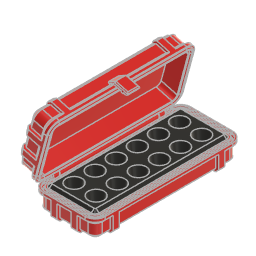
ER16 Collet Rugged Case (Autodesk Fusion 360 design; units mm, degrees)
Autodesk Fusion 360 part; units mm, degrees
note: some values were not read from the file. Chosen so that the rebuilt part matches the saved one: which face or edge a step refers to; where a step starts. Set by a fixed rule: which sketch regions a step uses.
sketch "Base Sketch" plane through (0, 0, 0) normal (0, 0, 1) x (1, 0, 0)
  line L0 (4, 0) -> (46, 0)
  line L1 (50, 4) -> (50, 131)
  line L2 (46, 135) -> (4, 135)
  line L3 (0, 131) -> (0, 4)
  arc A0 (46, 0) -> (50, 4) centre (46, 4) ccw
  arc A1 (50, 131) -> (46, 135) centre (46, 131) ccw
  arc A2 (4, 135) -> (0, 131) centre (4, 131) ccw
  arc A3 (0, 4) -> (4, 0) centre (4, 4) ccw
  point P0 (50, 0)
  point P1 (0, 135)
  dimension "d6" = 50
  dimension "d7" = 135
  dimension "d8" = 4
  constraint horizontal L0
  constraint vertical L1
  constraint horizontal L2
  constraint vertical L3
  constraint coincident P0 L0
  constraint coincident P0 L1
  constraint tangent L0 A0
  constraint tangent L1 A0
  constraint tangent L1 A1
  constraint tangent L2 A1
  constraint equal A0 A1
  constraint coincident P1 L2
  constraint coincident P1 L3
  constraint tangent L2 A2
  constraint tangent L3 A2
  constraint equal A0 A2
  constraint coincident origin L0
  constraint coincident origin L3
  constraint tangent L0 A3
  constraint tangent L3 A3
  constraint equal A0 A3
  measures "d6" distance of origin P0
  measures "d7" distance of origin P1
  measures "d8" radius of A0
ref_plane "WorkPlane1" through (0, 67.5, 0) normal (0, 1, 0) x (0, 0, 1)
sketch "Top Sketch" plane through (0, 67.5, 0) normal (0, 1, 0) x (1, 0, 0)
  line L0 (0, 0) -> (-3, 0)
  line L1 (-3, 0) -> (-3, -16.5)
  line L2 (-3, -16.5) -> (0, -16.5)
  line L3 (0, -16.5) -> (0, 0)
  line L4 (-3, -16.5) -> (-6, -16.5)
  line L5 (-6, -16.5) -> (-6, -13.5)
  line L6 (-6, -13.5) -> (-3, -13.5)
  line L7 (-3, -13.5) -> (-3, -16.5)
  line L8 (0, 0) -> (25, 0)
  line L9 (25, 0) -> (25, 3)
  line L10 (25, 3) -> (0, 3)
  line L11 (0, 3) -> (0, 0)
  line L12 (0, 3) -> (-3, 0)
  line L13 (-6, -13.5) -> (-3, -10.5)
  line L14 (-4.5, -16.5) -> (-3.3536, -17.6464)
  line L15 (-4.5, -16.5) -> (-2.3787, -16.5) construction
  line L16 (-2.6464, -17.6464) -> (-1.5, -16.5)
  arc A0 (-3.3536, -17.6464) -> (-2.6464, -17.6464) centre (-3, -17.2929) ccw
  dimension "d12" = 3
  dimension "d13" = 16.5
  dimension "d14" = 3
  dimension "d15" = 3
  dimension "d16" = 25
  dimension "d17" = 3
  dimension "d97" = 45
  dimension "d146" = 0.5
  dimension "d284" = 45
  constraint horizontal L0
  constraint vertical L1
  constraint horizontal L2
  constraint vertical L3
  constraint coincident L0.start L3.end
  constraint horizontal L4
  constraint vertical L5
  constraint horizontal L6
  constraint vertical L7
  constraint horizontal L8
  constraint vertical L9
  constraint horizontal L10
  constraint vertical L11
  constraint coincident L1 L13.end
  constraint parallel L12 L13
  constraint horizontal L15
  constraint midpoint L4 L14.start
  constraint midpoint L2 L16.end
  constraint tangent L14 A0
  constraint tangent L16 A0
  measures "d12" distance of L0.start L0.end
  measures "d13" distance of L0.start L2.end
  measures "d14" distance of L1.end L4.end
  measures "d15" distance of L1.end L6.end
  measures "d16" distance of L0.start L8.end
  measures "d17" distance of L0.start L10.end
  measures "d97" angle of L14 L15
  measures "d146" radius of A0
  measures "d284" angle of L2 L16
sweep "Sweep1" add profiles "Top Sketch" path "Base Sketch" along L0 A0 L1 A1 L2 A2 L3 A3 section 1 contours L0 L1 L2 L3 L7 | L8 L9 L10 L11 | L0 L11 L12 | L1 L6 L13 | L1 L4 L5 L6 L7 makes body 1
sketch "Bottom Sketch" plane through (0, 67.5, 0) normal (0, 1, 0) x (1, 0, 0)
  line L0 (0, 0) -> (-3, 0)
  line L1 (-3, 0) -> (-3, -16.5)
  line L2 (-3, -16.5) -> (0, -16.5)
  line L3 (0, -16.5) -> (0, 0)
  line L4 (0, 0) -> (25, 0)
  line L5 (25, 0) -> (25, 3)
  line L6 (25, 3) -> (0, 3)
  line L7 (0, 3) -> (0, 0)
  line L8 (-3, -16.5) -> (-6, -16.5)
  line L9 (-6, -16.5) -> (-6, -13.5)
  line L10 (-6, -13.5) -> (-3, -13.5)
  line L11 (-3, -13.5) -> (-3, -16.5)
  line L12 (0, 3) -> (-3, 0)
  line L13 (-6, -13.5) -> (-3, -10.5)
  line L14 (-4.5, -16.5) -> (-1.5, -16.5)
  line L15 (-1.5, -16.5) -> (-1.5, -13.5)
  line L16 (-1.5, -13.5) -> (-4.5, -13.5)
  line L17 (-4.5, -13.5) -> (-4.5, -16.5)
  line L18 (-3.3536, -13.8536) -> (-4.5, -15)
  line L19 (-2.6464, -13.8536) -> (-1.5, -15)
  arc A0 (-2.6464, -13.8536) -> (-3.3536, -13.8536) centre (-3, -14.2071) ccw
  dimension "d24" = 3
  dimension "d25" = 16.5
  dimension "d26" = 25
  dimension "d27" = 3
  dimension "d28" = 3
  dimension "d29" = 3
  dimension "d90" = 3
  dimension "d145" = 0.5
  constraint horizontal L0
  constraint vertical L1
  constraint horizontal L2
  constraint vertical L3
  constraint coincident L0.start L3.end
  constraint horizontal L4
  constraint vertical L5
  constraint horizontal L6
  constraint vertical L7
  constraint horizontal L8
  constraint vertical L9
  constraint horizontal L10
  constraint vertical L11
  constraint coincident L1 L13.end
  constraint parallel L12 L13
  constraint horizontal L14
  constraint vertical L15
  constraint horizontal L16
  constraint vertical L17
  constraint midpoint L8 L14.start
  constraint midpoint L17 L18.end
  constraint midpoint L15 L19.end
  constraint perpendicular L18 L19
  constraint coincident L10.end L18
  constraint coincident L10.end L19
  constraint tangent L18 A0
  constraint tangent L19 A0
  measures "d24" distance of L0.start L0.end
  measures "d25" distance of L0.start L2.end
  measures "d26" distance of L0.start L4.end
  measures "d27" distance of L0.start L6.end
  measures "d28" distance of L1.end L8.end
  measures "d29" distance of L1.end L10.end
  measures "d90" distance of L14.start L16.end
  measures "d145" radius of A0
sweep "Sweep2" add profiles "Bottom Sketch" path "Base Sketch" along L0 A0 L1 A1 L2 A2 L3 A3 section 1 separate body makes body 2
ref_plane "WorkPlane2" through (0, 18, 0) normal (0, 1, 0) x (0, 0, 1)
sketch "Rib Bottom" plane through (0, 18, 0) normal (0, 1, 0) x (1, 0, 0)
  line L0 (0, 0) -> (-6, 0)
  line L1 (-6, 0) -> (-6, -16.5)
  line L2 (-6, -16.5) -> (0, -16.5)
  line L3 (0, -16.5) -> (0, 0)
  line L4 (0, 0) -> (25, 0)
  line L5 (25, 0) -> (25, 3)
  line L6 (25, 3) -> (0, 3)
  line L7 (0, 3) -> (0, 0)
  line L8 (0, 0) -> (-3, 0)
  line L9 (-3, 0) -> (-3, 3)
  line L10 (-3, 3) -> (0, 3)
  line L11 (0, 3) -> (0, 0)
  line L12 (-3, 3) -> (-6, 0)
  dimension "d37" = 6
  dimension "d38" = 16.5
  dimension "d39" = 25
  dimension "d40" = 3
  dimension "d41" = 3
  dimension "d42" = 3
  constraint horizontal L0
  constraint vertical L1
  constraint horizontal L2
  constraint vertical L3
  constraint coincident L0.start L3.end
  constraint horizontal L4
  constraint vertical L5
  constraint horizontal L6
  constraint vertical L7
  constraint horizontal L8
  constraint vertical L9
  constraint horizontal L10
  constraint vertical L11
  measures "d37" distance of L0.start L0.end
  measures "d38" distance of L0.start L2.end
  measures "d39" distance of L0.start L4.end
  measures "d40" distance of L0.start L6.end
  measures "d41" distance of L0.start L8.end
  measures "d42" distance of L0.start L6.end
extrude "Extrude1" add sketch "Rib Bottom" against normal blind 6 bodies 2
ref_plane "WorkPlane3" through (0, 117, 0) normal (0, 1, 0) x (0, 0, 1)
extrude "Extrude2" add sketch "Rib Bottom" along normal blind 6 from surface at 99 bodies 2
ref_plane "WorkPlane4" through (25, 0, 0) normal (1, 0, 0) x (0, 1, 0)
mirror "Mirror1" about plane through (25, 0, 0) normal (1, 0, 0) of "Extrude1", "Extrude2"
sketch "Rib Top" plane through (0, 67.5, 0) normal (0, 1, 0) x (1, 0, 0)
  line L0 (0, 0) -> (-6, 0)
  line L1 (-6, 0) -> (-6, -16.5)
  line L2 (-6, -16.5) -> (0, -16.5)
  line L3 (0, -16.5) -> (0, 0)
  line L4 (0, 0) -> (25, 0)
  line L5 (25, 0) -> (25, 3)
  line L6 (25, 3) -> (0, 3)
  line L7 (0, 3) -> (0, 0)
  line L8 (0, 0) -> (-3, 0)
  line L9 (-3, 0) -> (-3, 3)
  line L10 (-3, 3) -> (0, 3)
  line L11 (0, 3) -> (0, 0)
  line L12 (-3, 3) -> (-6, 0)
  dimension "d52" = 6
  dimension "d53" = 16.5
  dimension "d54" = 25
  dimension "d55" = 3
  dimension "d56" = 3
  dimension "d57" = 3
  constraint horizontal L0
  constraint vertical L1
  constraint horizontal L2
  constraint vertical L3
  constraint coincident L0.start L3.end
  constraint horizontal L4
  constraint vertical L5
  constraint horizontal L6
  constraint vertical L7
  constraint horizontal L8
  constraint vertical L9
  constraint horizontal L10
  constraint vertical L11
  measures "d52" distance of L0.start L0.end
  measures "d53" distance of L0.start L2.end
  measures "d54" distance of L0.start L4.end
  measures "d55" distance of L0.start L6.end
  measures "d56" distance of L0.start L8.end
  measures "d57" distance of L0.start L6.end
extrude "Extrude3" add sketch "Rib Top" against normal blind 6 from surface at -49.5 bodies 1
extrude "Extrude4" add sketch "Rib Top" along normal blind 6 from surface at 49.5 bodies 1
mirror "Mirror2" about plane through (25, 0, 0) normal (1, 0, 0) of "Extrude3", "Extrude4"
ref_plane "WorkPlane5" through (18, 0, 0) normal (1, 0, 0) x (0, 1, 0)
ref_plane "WorkPlane6" through (32, 0, 0) normal (1, 0, 0) x (0, 1, 0)
sketch "Rib Wid" plane through (18, 0, 0) normal (1, 0, 0) x (0, 1, 0)
  line L0 (0, 0) -> (-6, 0)
  line L1 (-6, 0) -> (-6, 16.5)
  line L2 (-6, 16.5) -> (0, 16.5)
  line L3 (0, 16.5) -> (0, 0)
  line L4 (0, 0) -> (67.5, 0)
  line L5 (67.5, 0) -> (67.5, -3)
  line L6 (67.5, -3) -> (0, -3)
  line L7 (0, -3) -> (0, 0)
  line L8 (0, 0) -> (-3, 0)
  line L9 (-3, 0) -> (-3, -3)
  line L10 (-3, -3) -> (0, -3)
  line L11 (0, -3) -> (0, 0)
  line L12 (-3, -3) -> (-6, 0)
  line L13 (0, -3) -> (-6, -3)
  line L14 (-6, -3) -> (-6, 13.5)
  line L15 (-6, 13.5) -> (0, 13.5)
  line L16 (0, 13.5) -> (0, -3)
  dimension "d68" = 6
  dimension "d69" = 16.5
  dimension "d70" = 67.5
  dimension "d71" = 3
  dimension "d72" = 3
  dimension "d73" = 3
  dimension "d74" = 6
  dimension "d75" = 16.5
  constraint horizontal L0
  constraint vertical L1
  constraint horizontal L2
  constraint vertical L3
  constraint coincident L0.start L3.end
  constraint horizontal L4
  constraint vertical L5
  constraint horizontal L6
  constraint vertical L7
  constraint horizontal L8
  constraint vertical L9
  constraint horizontal L10
  constraint vertical L11
  constraint horizontal L13
  constraint vertical L14
  constraint horizontal L15
  constraint vertical L16
  measures "d68" distance of L0.start L0.end
  measures "d69" distance of L0.start L2.end
  measures "d70" distance of L0.start L4.end
  measures "d71" distance of L0.start L6.end
  measures "d72" distance of L0.start L8.end
  measures "d73" distance of L0.start L6.end
  measures "d74" distance of L6.end L13.end
  measures "d75" distance of L6.end L15.end
extrude "Extrude5" add sketch "Rib Wid" against normal blind 6 contours L0 L7 L8 L9 L10 L11 L13 L16 | L0 L1 L3 L8 L14 L15 L16 | L4 L5 L6 L7 L11 L16 | L0 L9 L12 | L1 L2 L3 L15 bodies 2
extrude "Extrude6" add sketch "Rib Wid" along normal blind 6 from surface at 14 contours L0 L7 L8 L9 L10 L11 L13 L16 | L0 L1 L3 L8 L14 L15 L16 | L4 L5 L6 L7 L11 L16 | L0 L9 L12 | L1 L2 L3 L15 bodies 2
ref_plane "WorkPlane7" through (25, 67.5, 5.25) normal (0, -1, 0) x (0, 0, -1)
mirror "Mirror3" about plane through (25, 67.5, 5.25) normal (0, -1, 0) of "Extrude5", "Extrude6"
extrude "Extrude7" add sketch "Rib Wid" against normal blind 6 contours L0 L7 L8 L9 L10 L11 L13 L16 | L0 L1 L3 L8 L14 L15 L16 | L4 L5 L6 L7 L11 L16 | L0 L9 L12 bodies 1
extrude "Extrude8" add sketch "Rib Wid" along normal blind 6 from surface at 14 contours L0 L7 L8 L9 L10 L11 L13 L16 | L0 L1 L3 L8 L14 L15 L16 | L4 L5 L6 L7 L11 L16 | L0 L9 L12 bodies 1
mirror "Mirror4" about plane through (25, 67.5, 5.25) normal (0, -1, 0) of "Extrude7", "Extrude8"
sweep "Sweep3" cut profiles "Bottom Sketch" path "Base Sketch" along L0 A0 L1 A1 L2 A2 L3 A3 section 1 contours L1 L2 L11 L14 L15 L19 A0 | L1 L8 L11 L14 L17 L18 A0 bodies 2
sweep "Sweep4" add profiles "Top Sketch" path "Base Sketch" along L0 A0 L1 A1 L2 A2 L3 A3 section 1 contours L2 L4 L14 L16 A0 bodies 1
sketch "Hinge" plane through (0, 0, 0) normal (0, 1, 0) x (1, 0, 0)
  line L0 (0, 0) -> (-6, 0) construction
  line L1 (-6, 0) -> (-6, -16.5) construction
  line L2 (-6, -16.5) -> (0, -16.5) construction
  line L3 (0, -16.5) -> (0, 0) construction
  circle A0 centre (-6, -16.5) radius 3
  circle A1 centre (-6, -16.5) radius 1.5
  circle A2 centre (-6, -16.5) radius 3.1
  line L4 (-6, -16.5) -> (-4.5, -16.5)
  line L5 (-4.5, -16.5) -> (-4.5, -19.5)
  line L6 (-4.5, -19.5) -> (-6, -19.5)
  line L7 (-6, -19.5) -> (-6, -16.5)
  line L8 (-6, -16.5) -> (-7.5, -16.5)
  line L9 (-7.5, -16.5) -> (-7.5, -19.5)
  line L10 (-7.5, -19.5) -> (-6, -19.5)
  line L11 (-6, -19.5) -> (-6, -16.5)
  line L12 (0, 0) -> (-6, 0) construction
  line L13 (-6, 0) -> (-6, -16.5) construction
  line L14 (-6, -16.5) -> (0, -16.5) construction
  line L15 (0, -16.5) -> (0, 0) construction
  circle A3 centre (-6, -16.5) radius 3
  circle A4 centre (-6, -16.5) radius 3.2
  dimension "d329" = 6
  dimension "d330" = 16.5
  dimension "d331" = 6
  dimension "d332" = 3
  dimension "d339" = 6.2
  dimension "d345" = 1.5
  dimension "d346" = 3
  dimension "d347" = 1.5
  dimension "d348" = 3
  dimension "d355" = 6
  dimension "d356" = 16.5
  dimension "d357" = 6
  dimension "d358" = 0.2
  constraint horizontal L0
  constraint vertical L1
  constraint horizontal L2
  constraint vertical L3
  constraint coincident L0.start L3.end
  constraint coincident L1.end L2.start
  constraint concentric A0 A1
  constraint concentric A0 A2
  constraint horizontal L4
  constraint vertical L5
  constraint horizontal L6
  constraint vertical L7
  constraint horizontal L8
  constraint vertical L9
  constraint horizontal L10
  constraint vertical L11
  constraint horizontal L12
  constraint vertical L13
  constraint horizontal L14
  constraint vertical L15
  measures "d329" distance of L0.start L0.end
  measures "d330" distance of L0.start L2.end
  measures "d331" diameter of A0
  measures "d332" diameter of A1
  measures "d339" diameter of A2
  measures "d345" distance of L1.end L4.end
  measures "d346" distance of L1.end L6.end
  measures "d347" distance of L1.end L8.end
  measures "d348" distance of L1.end L6.end
  measures "d355" distance of L0.start L0.end
  measures "d356" distance of L0.start L2.end
  measures "d357" diameter of A3
extrude "Extrude58" add sketch "Hinge" along normal up to surface (6 mm away) from surface at 12 contours A0 A1 L5 L9 A3 | A0 A1 L7 L9 L11 A3 | A0 A1 L5 L7 L11 A3 | A1 L7 L8 L11 | A1 L4 L8 | A1 L4 L7 L11 bodies 1
extrude "Extrude59" add sketch "Hinge" along normal up to surface (6 mm away) from surface at 117 contours A0 A1 L5 L9 A3 | A0 A1 L7 L9 L11 A3 | A0 A1 L5 L7 L11 A3 | A1 L7 L8 L11 | A1 L4 L8 | A1 L4 L7 L11 bodies 1
extrude "Extrude60" cut sketch "Hinge" along normal up to surface (99 mm away) from surface at 18 contours A0 A1 L5 L9 A3 | A0 A2 L5 L9 A3 | A0 A1 L7 L9 L11 A3 | A0 A2 L9 L10 A3 | A0 A2 L5 L6 A3 | A0 A1 L5 L7 L11 A3 | A2 L6 L10 | A1 L7 L8 L11 | A1 L4 L8 | A1 L4 L7 L11 bodies 1
extrude "Extrude61" cut sketch "Hinge" against normal blind 0.4 from surface at 18 contours A0 A1 L7 L9 L11 A3 | A0 A1 L5 L7 L11 A3 | A1 L7 L8 L11 | A1 L4 L7 L11 bodies 1
extrude "Extrude62" cut sketch "Hinge" along normal blind 0.4 from surface at 117 contours A0 A1 L7 L9 L11 A3 | A0 A1 L5 L7 L11 A3 | A1 L7 L8 L11 | A1 L4 L7 L11 bodies 1
extrude "Extrude63" cut sketch "Hinge" along normal up to surface (6.4 mm away) from surface at 11.8 contours A0 A1 L5 L9 A3 | A0 A2 L5 L9 A3 | A0 A1 L7 L9 L11 A3 | A0 A2 L9 L10 A3 | A0 A2 L5 L6 A3 | A0 A1 L5 L7 L11 A3 | A2 L6 L10 | A1 L7 L8 L11 | A1 L4 L8 | A2 L5 L9 A4 | A2 L9 L10 A4 | A1 L4 L7 L11 | A2 L5 L6 A4 | A2 L6 L10 A4 bodies 2
extrude "Extrude64" cut sketch "Hinge" along normal up to surface (6.4 mm away) from surface at 116.8 contours A0 A1 L5 L9 A3 | A0 A2 L5 L9 A3 | A0 A1 L7 L9 L11 A3 | A0 A2 L9 L10 A3 | A0 A2 L5 L6 A3 | A0 A1 L5 L7 L11 A3 | A2 L6 L10 | A1 L7 L8 L11 | A1 L4 L8 | A2 L5 L9 A4 | A2 L9 L10 A4 | A1 L4 L7 L11 | A2 L5 L6 A4 | A2 L6 L10 A4 bodies 2
extrude "Extrude65" add sketch "Hinge" along normal up to surface (98.6 mm away) from surface at 18.2 contours A0 A1 L5 L9 A3 | A0 A1 L7 L9 L11 A3 | A0 A1 L5 L7 L11 A3 | A1 L7 L8 L11 | A1 L4 L8 | A1 L4 L7 L11 bodies 2
sketch "Sketch16" plane through (0, 0, 0) normal (0, 1, 0) x (1, 0, 0)
  line L0 (0, 0) -> (50, 0) construction
  line L1 (50, 0) -> (50, -16.5) construction
  line L2 (50, -16.5) -> (0, -16.5) construction
  line L3 (0, -16.5) -> (0, 0) construction
  line L4 (50, 0) -> (51.5, 0) construction
  line L5 (51.5, 0) -> (51.5, -16.5) construction
  line L6 (51.5, -16.5) -> (50, -16.5) construction
  line L7 (50, -16.5) -> (50, 0) construction
  line L8 (51.5, -16.5) -> (54.5, -16.5)
  line L9 (54.5, -16.5) -> (54.5, -19.5)
  line L10 (54.5, -19.5) -> (51.5, -19.5)
  line L11 (51.5, -19.5) -> (51.5, -16.5)
  dimension "d370" = 50
  dimension "d371" = 16.5
  dimension "d372" = 1.5
  dimension "d373" = 16.5
  dimension "d374" = 3
  dimension "d375" = 3
  constraint horizontal L0
  constraint vertical L1
  constraint horizontal L2
  constraint vertical L3
  constraint coincident L0.start L3.end
  constraint horizontal L4
  constraint vertical L5
  constraint horizontal L6
  constraint vertical L7
  constraint horizontal L8
  constraint vertical L9
  constraint horizontal L10
  constraint vertical L11
  measures "d370" distance of L0.start L0.end
  measures "d371" distance of L0.start L2.end
  measures "d372" distance of L0.end L4.end
  measures "d373" distance of L0.end L1.end
  measures "d374" distance of L5.end L8.end
  measures "d375" distance of L5.end L10.end
sketch "Sketch17" plane through (0, 117, 0) normal (0, -1, 0) x (1, 0, 0)
  line L0 (-4.5, 19.0981) -> (-4.5, 16.5)
  line L1 (-4.5, 16.5) -> (-7.5, 16.5)
  line L2 (-7.5, 16.5) -> (-7.5, 19.0981)
  arc A0 (-7.5, 19.0981) -> (-6, 13.5) centre (-6, 16.5) ccw
  line L3 (-6, 13.5) -> (-6, 0)
  line L4 (-6, 0) -> (-3, -3)
  line L5 (-3, -3) -> (0, -3)
  line L6 (0, -3) -> (-3, 0)
  line L7 (-3, 0) -> (-3, 10.5)
  line L8 (-3, 10.5) -> (-5.9016, 13.4016)
  arc A1 (-5.9016, 13.4016) -> (-3.1691, 17.7634) centre (-6, 16.5) ccw
  arc A2 (-3.1691, 17.7634) -> (-3.2594, 17.7203) centre (-3, 17.2929) ccw
  circle A3 centre (-6, 16.5) radius 1.5
  arc A4 (-3.2594, 17.7203) -> (-4.5, 19.0981) centre (-6, 16.5) ccw
  dimension "d376" = 3
  constraint concentric A0 A3
  measures "d376" diameter of A3
revolve "Revolve1" cut sketch "Sketch17" angle 360 about axis through (-4.5, 117, 16.5) along (-1, 0, 0) contours L1 A3 picked at (-6.4131, 16.2183) bodies 1
sketch "Sketch18" plane through (0, 116.8, 0) normal (0, 1, 0) x (-1, 0, 0)
  line L0 (3.8787, 14.3787) -> (3.7373, 14.2373)
  arc A0 (3.7373, 14.2373) -> (5.8059, 13.3059) centre (6, 16.5) ccw
  line L1 (5.8059, 13.3059) -> (6, 13.5)
  arc A1 (6, 13.5) -> (3.8787, 14.3787) centre (6, 16.5) ccw
  circle A2 centre (6, 16.5) radius 1.5
  line L2 (6, 16.5) -> (4.5, 16.5)
  line L3 (6, 16.5) -> (6.2, 16.5)
  line L4 (6.2, 16.5) -> (7.5, 16.5)
  dimension "d378" = 3
  constraint concentric A0 A2
  constraint coincident A0.centre A1.centre
  constraint coincident A2 L2.end
  constraint horizontal L2
  constraint parallel L2 L3
  constraint coincident A2 L4.end
  constraint parallel L2 L4
  measures "d378" diameter of A2
revolve "Revolve2" add sketch "Sketch18" angle 360 about axis through (-6.2, 116.8, 16.5) along (-1, 0, 0) contours A2 L2 L3 L4 picked at (5.1364, 16.0014) bodies 2
sketch "Sketch19" plane through (0, 18.2, 0) normal (0, -1, 0) x (1, 0, 0)
  arc A0 (-3.8787, 14.3787) -> (-6, 13.5) centre (-6, 16.5) ccw
  line L0 (-6, 13.5) -> (-5.8059, 13.3059)
  arc A1 (-5.8059, 13.3059) -> (-3.7373, 14.2373) centre (-6, 16.5) ccw
  line L1 (-3.7373, 14.2373) -> (-3.8787, 14.3787)
  circle A2 centre (-6, 16.5) radius 1.5
  line L2 (-6, 16.5) -> (-4.5, 16.5)
  line L3 (-6, 16.5) -> (-7.5, 16.5)
  dimension "d380" = 3
  constraint concentric A0 A2
  constraint coincident A0.centre A1.centre
  constraint coincident A2 L2.end
  constraint horizontal L2
  constraint coincident A2 L3.end
  constraint parallel L2 L3
  measures "d380" diameter of A2
revolve "Revolve3" add sketch "Sketch19" angle 360 about axis through (-6, 18.2, 16.5) along (1, 0, 0) contours A2 L2 L3 picked at (-5.0056, 16.4255) bodies 2
sketch "Sketch20" plane through (0, 18, 0) normal (0, 1, 0) x (-1, 0, 0)
  line L0 (4.5, 16.5) -> (4.5, 19.0981)
  arc A0 (4.5, 19.0981) -> (3.2594, 17.7203) centre (6, 16.5) ccw
  arc A1 (3.2594, 17.7203) -> (3.1691, 17.7634) centre (3, 17.2929) ccw
  arc A2 (3.1691, 17.7634) -> (5.9016, 13.4016) centre (6, 16.5) ccw
  line L1 (5.9016, 13.4016) -> (3, 10.5)
  line L2 (3, 10.5) -> (3, 0)
  line L3 (3, 0) -> (0, -3)
  line L4 (0, -3) -> (3, -3)
  line L5 (3, -3) -> (6, 0)
  line L6 (6, 0) -> (6, 13.5)
  arc A3 (6, 13.5) -> (7.5, 19.0981) centre (6, 16.5) ccw
  line L7 (7.5, 19.0981) -> (7.5, 16.5)
  line L8 (7.5, 16.5) -> (4.5, 16.5)
  circle A4 centre (6, 16.5) radius 1.5
  dimension "d382" = 3
  constraint concentric A0 A4
  measures "d382" diameter of A4
revolve "Revolve4" cut sketch "Sketch20" angle 360 about axis through (-7.5, 18, 16.5) along (1, 0, 0) contours L8 A4 picked at (6.0318, 15.9269) bodies 1
chamfer "Chamfer10" distance 0.39 angle 45 4 edges at (-4.5, 117.4, 17.799) (-7.5, 117.4, 17.799) (-4.5, 17.6, 17.799) (-7.5, 17.6, 17.799) on bodies 1
sketch "Latch" plane through (0, 0, 0) normal (0, 1, 0) x (1, 0, 0)
  line L0 (0, 0) -> (53, 0) construction
  line L1 (53, 0) -> (53, -16.5) construction
  line L2 (53, -16.5) -> (0, -16.5) construction
  line L3 (0, -16.5) -> (0, 0) construction
  line L4 (0, 0) -> (53, 0) construction
  line L5 (53, 0) -> (53, -16.5)
  line L6 (53, -16.5) -> (0, -16.5) construction
  line L7 (0, -16.5) -> (0, 0) construction
  line L8 (53, -16.5) -> (56, -16.5) construction
  line L9 (56, -16.5) -> (56, -13.5) construction
  line L10 (56, -13.5) -> (53, -13.5) construction
  line L11 (53, -13.5) -> (53, -16.5) construction
  line L12 (53, -16.5) -> (56, -16.5) construction
  line L13 (56, -16.5) -> (56, -13.5) construction
  line L14 (56, -13.5) -> (53, -13.5) construction
  line L15 (53, -13.5) -> (53, -16.5) construction
  line L16 (53, -13.5) -> (56, -13.5)
  line L17 (56, -13.5) -> (56, -10.5)
  line L18 (56, -10.5) -> (53, -10.5)
  line L19 (53, -10.5) -> (53, -13.5)
  line L20 (53, -13.5) -> (56, -13.5)
  line L21 (56, -13.5) -> (56, -10.5)
  line L22 (56, -10.5) -> (53, -10.5)
  line L23 (53, -10.5) -> (53, -13.5)
  line L24 (56, -13.5) -> (59, -13.5)
  line L25 (59, -13.5) -> (59, -22)
  line L26 (59, -22) -> (56, -22)
  line L27 (56, -22) -> (56, -13.5)
  line L28 (53, -16.5) -> (56, -16.5)
  line L29 (56, -16.5) -> (56, -19.5)
  line L30 (56, -19.5) -> (53, -19.5)
  line L31 (53, -19.5) -> (53, -16.5)
  line L32 (59, -13.5) -> (56, -10.5)
  circle A0 centre (56, -22) radius 2
  line L33 (56, -10.5) -> (53, -7.5)
  line L34 (56, -10.5) -> (80.2426, -10.5) construction
  dimension "d385" = 53
  dimension "d386" = 16.5
  dimension "d387" = 53
  dimension "d388" = 16.5
  dimension "d389" = 3
  dimension "d390" = 3
  dimension "d391" = 3
  dimension "d392" = 3
  dimension "d393" = 3
  dimension "d394" = 3
  dimension "d395" = 3
  dimension "d396" = 3
  dimension "d397" = 3
  dimension "d398" = 8.5
  dimension "d399" = 3
  dimension "d400" = 3
  dimension "d401" = 4
  dimension "d402" = 135
  constraint horizontal L0
  constraint vertical L1
  constraint horizontal L2
  constraint vertical L3
  constraint coincident L0.start L3.end
  constraint horizontal L4
  constraint vertical L5
  constraint horizontal L6
  constraint vertical L7
  constraint horizontal L8
  constraint vertical L9
  constraint horizontal L10
  constraint vertical L11
  constraint horizontal L12
  constraint vertical L13
  constraint horizontal L14
  constraint vertical L15
  constraint horizontal L16
  constraint vertical L17
  constraint horizontal L18
  constraint vertical L19
  constraint horizontal L20
  constraint vertical L21
  constraint horizontal L22
  constraint vertical L23
  constraint horizontal L24
  constraint vertical L25
  constraint horizontal L26
  constraint vertical L27
  constraint horizontal L28
  constraint vertical L29
  constraint horizontal L30
  constraint vertical L31
  constraint horizontal L34
  constraint coincident L1 L33.end
  constraint coincident L26.end L27.start
  measures "d385" distance of L0.start L0.end
  measures "d386" distance of L0.start L2.end
  measures "d387" distance of L0.start L0.end
  measures "d388" distance of L0.start L2.end
  measures "d389" distance of L1.end L8.end
  measures "d390" distance of L1.end L10.end
  measures "d391" distance of L1.end L8.end
  measures "d392" distance of L1.end L10.end
  measures "d393" distance of L10.end L9.end
  measures "d394" distance of L10.end L18.end
  measures "d395" distance of L10.end L9.end
  measures "d396" distance of L10.end L18.end
  measures "d397" distance of L9.end L24.end
  measures "d398" distance of L9.end L26.end
  measures "d399" distance of L1.end L8.end
  measures "d400" distance of L1.end L30.end
  measures "d401" diameter of A0
  measures "d402" angle of L33 L34
extrude "Extrude66" add sketch "Latch" along normal mid plane 12 from surface at 67.5 contours L5 L18 L22 L33 | L5 L16 L17 L18 L19 L20 L21 L22 L23 | L17 L21 L24 L32 | L24 L25 L26 L27 L29 A0 | L26 L27 A0 | L26 L27 A0 bodies 1
extrude "Extrude67" cut sketch "Latch" along normal mid plane 12.8 from surface at 67.5 contours L5 L16 L17 L18 L19 L20 L21 L22 L23 bodies 2
chamfer "Chamfer11" distance 2 angle 45 2 edges at (54.5, 73.9, 12) (54.5, 61.1, 12) on bodies 2
chamfer "Chamfer12" distance 1 angle 45 4 edges at (54.5858, 61.5, 23.4142) (59, 61.5, 17.75) (54.5858, 73.5, 23.4142) (59, 73.5, 17.75) on bodies 1
chamfer "Chamfer13" distance 1 angle 45 4 edges at (55.5001, 61.5, 10.0001) (55.5001, 73.5, 10.0001) (58.5001, 61.9999, 13.0001) (58.5001, 73.0001, 13.0001) on bodies 1
sketch "Sketch22" plane through (0, 61.5, 0) normal (0, -1, 0) x (1, 0, 0)
  line L0 (53, 8.9142) -> (58, 13.9142)
  line L1 (58, 13.9142) -> (58, 22)
  arc A0 (57, 22) -> (56, 21) centre (56, 22) ccw
  line L2 (56, 21) -> (56, 16.5)
  line L3 (56, 16.5) -> (56, 13.5)
  line L4 (56, 13.5) -> (53, 10.5)
  line L5 (56, 21) -> (59, 21)
  line L6 (59, 21) -> (59, 27)
  line L7 (59, 27) -> (56, 27)
  line L8 (56, 27) -> (56, 21)
  line L9 (58, 22) -> (57, 22)
  line L10 (53, 10.5) -> (53, 8.9142)
  dimension "d412" = 3
  dimension "d413" = 6
  constraint horizontal L5
  constraint vertical L6
  constraint horizontal L7
  constraint vertical L8
  constraint coincident A0.end L2.start
  measures "d412" distance of A0.end L5.end
  measures "d413" distance of A0.end L7.end
extrude "Extrude68" add sketch "Sketch22" against normal blind 12 contours L1 A0 L5 L8 L9 | L1 A0 L5 L6 L7 L8 L9 bodies 1
chamfer "Chamfer14" distance 1 angle 45 2 edges at (59, 61.5, 24) (59, 73.5, 24) on bodies 1
chamfer "Chamfer15" distance 1 angle 45 2 edges at (59, 67.5, 27) (56, 67.5, 27) on bodies 1
copy_body "Body->Comp1" bodies 1 removing the originals makes body 3 in component "Paramatric-Top-Case"
copy_body "Body->Comp2" bodies 2 removing the originals makes body 4 in component "Parametric-Bottom-Case"
sketch "Sketch23" plane through (0, 0, 0) normal (0, 0, 1) x (-1, 0, 0)
  line L0 (-46, -135) -> (-4, -135)
  arc A0 (-4, -135) -> (0, -131) centre (-4, -131) ccw
  line L1 (0, -131) -> (0, -4)
  arc A1 (0, -4) -> (-4, 0) centre (-4, -4) ccw
  line L2 (-4, 0) -> (-46, 0)
  arc A2 (-46, 0) -> (-50, -4) centre (-46, -4) ccw
  line L3 (-50, -4) -> (-50, -131)
  arc A3 (-50, -131) -> (-46, -135) centre (-46, -131) ccw
  circle A4 centre (-14, -15) radius 7.85
  line L4 (-14, -15) -> (-36.6683, -15)
  line L5 (-36.6683, -15) -> (-14, -15)
  line L6 (-14, -15) -> (-14, -35.3607)
  circle A5 centre (-36, -15) radius 7.85
  circle A6 centre (-14, -36) radius 7.85
  circle A7 centre (-36, -36) radius 7.85
  circle A8 centre (-14, -57) radius 7.85
  circle A9 centre (-36, -57) radius 7.85
  circle A10 centre (-14, -78) radius 7.85
  circle A11 centre (-36, -78) radius 7.85
  circle A12 centre (-14, -99) radius 7.85
  circle A13 centre (-36, -99) radius 7.85
  circle A14 centre (-14, -120) radius 7.85
  circle A15 centre (-36, -120) radius 7.85
  line L7 (-0.1, -131) -> (-0.1, -4)
  arc A16 (-0.1, -4) -> (-4, -0.1) centre (-4, -4) ccw
  line L8 (-4, -0.1) -> (-46, -0.1)
  arc A17 (-46, -0.1) -> (-49.9, -4) centre (-46, -4) ccw
  line L9 (-49.9, -4) -> (-49.9, -131)
  arc A18 (-49.9, -131) -> (-46, -134.9) centre (-46, -131) ccw
  line L10 (-46, -134.9) -> (-4, -134.9)
  arc A19 (-4, -134.9) -> (-0.1, -131) centre (-4, -131) ccw
  dimension "d423" = 15.7
  dimension "d426" = -22
  dimension "d427" = -21
  dimension "d428" = -0.1
  dimension "d429" = 13.9
  dimension "d430" = 13.9
  dimension "d431" = 14.9
  dimension "d432" = 14.9
  constraint coincident A4.centre L4.start
  constraint horizontal L4
  constraint perpendicular L5 L6
  measures "d423" diameter of A4
  measures "d429" distance of A14.centre L7
  measures "d430" distance of A15.centre L9
  measures "d431" distance of A4.centre L8
  measures "d432" distance of A14.centre L10
extrude "Extrude1'" add sketch "Sketch23" along normal blind 19 separate body contours A4 L4 L5 L6 | A4 L4 L5 L6 | A5 | A6 | A7 | A8 | A9 | A10 | A11 | A12 | A13 | A14 | A15 | L7 A16 L8 A17 L9 A18 L10 A19 makes body 5 in component "ER16-Collet-Insert"
extrude "Extrude2'" cut sketch "Sketch23" against normal blind 14 draft -7.9 from surface at 19 contours A4 L4 L5 L6 | A4 L4 L5 L6 | A5 | A6 | A7 | A8 | A9 | A10 | A11 | A12 | A13 | A14 | A15 bodies 5 in component "ER16-Collet-Insert"
chamfer "Chamfer1" distance 3 distance2 2.5 8 edges at (49.9, 67.5, 19) (48.7577, 133.7577, 19) (25, 134.9, 19) (1.2423, 133.7577, 19) (0.1, 67.5, 19) (1.2423, 1.2423, 19) (25, 0.1, 19) (48.7577, 1.2423, 19) measured on face at (28.0844, 132.4844, 19) measured on face at (28.0844, 132.4844, 19) measured on face at (28.0844, 132.4844, 19) measured on face at (28.0844, 132.4844, 19) measured on face at (28.0844, 132.4844, 19) measured on face at (28.0844, 132.4844, 19) measured on face at (28.0844, 132.4844, 19) measured on face at (28.0844, 132.4844, 19) on bodies 5 in component "ER16-Collet-Insert"
component "Paramatric-Top-Case" placed x (0.260661, 0, 0.96543) y (0, -1, 0) z (0.96543, 0, -0.260661) at (-20.3656, 135, 26.5935)
component "Parametric-Bottom-Case" placed x (1, 0, 0) y (0, 1, 0) z (0, 0, 1) at (0, 0, 0)
component "ER16-Collet-Insert" placed x (1, 0, 0) y (0, 1, 0) z (0, 0, 1) at (0, 0, 0)
equation "len = 135 mm" comment "Min 50mm"
equation "wid = 50 mm" comment "Min 30mm"
equation "hei = 33 mm" comment "Min 15mm if split .5; Min 30 if split .25"
equation "shell = 3 mm" comment "Don't change. This is used in a lot of calculations"
equation "fillet = 4 mm" comment "Controls curvature of corners"
equation "d6 = wid"
equation "d7 = len"
equation "d8 = fillet"
equation "d9 = len / 2"
equation "splitTop = hei * 0.5" comment "Determines % of internal dimensions is within the lid"
equation "splitBottom = hei - splitTop" comment "Don't change"
equation "d12 = shell"
equation "d13 = splitTop"
equation "d14 = shell"
equation "d15 = shell"
equation "d16 = wid / 2"
equation "d17 = shell"
equation "d24 = shell"
equation "d25 = splitBottom"
equation "d26 = wid / 2"
equation "d27 = shell"
equation "d28 = shell"
equation "d29 = shell"
equation "d36 = shell * 6"
equation "d37 = shell * 2"
equation "d38 = splitBottom"
equation "d39 = wid / 2"
equation "d40 = shell"
equation "d41 = shell"
equation "d42 = shell"
equation "d43 = -shell * 2"
equation "d45 = len - ( shell * 6 )"
equation "d47 = shell * 2"
equation "d49 = wid / 2"
equation "d52 = shell * 2"
equation "d53 = splitTop"
equation "d54 = wid / 2"
equation "d55 = shell"
equation "d56 = shell"
equation "d57 = shell"
equation "d59 = -shell * 2"
equation "d62 = shell * 2"
equation "d66 = shell * 6"
equation "d67 = wid - ( shell * 6 )"
equation "d68 = shell * 2"
equation "d69 = splitBottom"
equation "d70 = len / 2"
equation "d71 = shell"
equation "d72 = shell"
equation "d73 = shell"
equation "d74 = shell * 2"
equation "d75 = splitTop"
equation "d76 = -shell * 2"
equation "d79 = shell * 2"
equation "d83 = -shell * 2"
equation "d86 = shell * 2"
equation "d90 = shell"
equation "clearance = 0.2 mm" comment "Don't change"
equation "d329 = shell * 2"
equation "d330 = splitTop"
equation "d331 = shell * 2"
equation "d332 = shell"
equation "d339 = shell * 2 + clearance"
equation "d345 = shell / 2"
equation "d346 = shell"
equation "d347 = shell / 2"
equation "d348 = shell"
equation "d350 = -clearance * 2"
equation "d353 = clearance * 2"
equation "d355 = shell * 2"
equation "d356 = splitBottom"
equation "d357 = shell * 2"
equation "d358 = clearance"
equation "d359 = clearance"
equation "d360 = clearance"
equation "d362 = clearance"
equation "d363 = clearance"
equation "d370 = wid"
equation "d371 = splitTop"
equation "d372 = shell / 2"
equation "d373 = splitTop"
equation "d374 = shell"
equation "d375 = shell"
equation "d376 = shell"
equation "d378 = shell"
equation "d380 = shell"
equation "d382 = shell"
equation "d385 = wid + shell"
equation "d386 = splitTop"
equation "d387 = wid + shell"
equation "d388 = splitBottom"
equation "d389 = shell"
equation "d390 = shell"
equation "d391 = shell"
equation "d392 = shell"
equation "d393 = shell"
equation "d394 = shell"
equation "d395 = shell"
equation "d396 = shell"
equation "d397 = shell"
equation "d398 = shell * 3 - 0.5 mm"
equation "d399 = shell"
equation "d400 = shell"
equation "d401 = shell * 2 - 2 mm"
equation "d404 = shell * 2"
equation "d407 = shell * 2 + ( clearance * 2 )"
equation "d412 = shell"
equation "d413 = shell * 2"
equation "d421 = -clearance"
equation "d429 = 8.5 mm + 5.4 mm"
equation "d431 = 8.5 mm + 6.4 mm"
named bodies: "Top", "Bottom"
